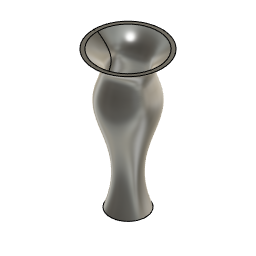
Vase v2 (Autodesk Fusion 360 design; units mm, degrees)
Autodesk Fusion 360 part; units mm, degrees
sketch "S-Vase-1" plane through (0, 0, 0) normal (0, 1, 0) x (1, 0, 0)
  line L0 (-88.461091, -147.362553) -> (-98.372625, -147.362553)
  spline S0 degree 5 poles (-98.372625, -147.362553) (-90.575572, -142.36067) (-76.825516, -132.431886) (-61.732191, -117.763849) (-51.958026, -98.828036) (-52.930643, -77.034995) (-62.024, -57.890704) (-74.243788, -41.693247) (-86.035966, -27.652867) (-95.531073, -13.982558) (-101.865459, 1.426054) (-104.795967, 20.4963) (-104.240926, 44.41601) (-100.243032, 73.849599) (-92.907373, 109.081445) (-82.364022, 150.155399) (-71.459298, 187.620816) (-61.929932, 218.259655) (-54.980996, 239.806153) (-51.35752, 250.859554) knots 0 0 0 0 0 0 0.06666667 0.13333333 0.2 0.26666667 0.33333333 0.4 0.46666667 0.53333333 0.6 0.66666667 0.73333333 0.8 0.86666667 0.93333333 1 1 1 1 1 1
  line L1 (-51.35752, 250.859554) -> (-0.678901, 250.859554)
  line L2 (-0.678901, 250.859554) -> (-0.453754, -147.362553)
  line L3 (-163.094718, -188.882386) -> (-33.650533, -105.84272)
  spline S1 degree 5 poles (-88.461091, -147.362553) (-80.720692, -142.397014) (-67.056368, -132.540065) (-52.008939, -117.977208) (-42.150348, -99.17113) (-42.881833, -77.499276) (-51.719986, -58.420857) (-63.770855, -42.243259) (-75.506283, -28.237163) (-85.061193, -14.682918) (-91.56478, 0.467783) (-94.773244, 19.11565) (-94.60872, 42.45327) (-91.110969, 71.147147) (-84.381692, 105.488788) (-74.546413, 145.528366) (-64.286411, 182.055738) (-55.283352, 211.930616) (-48.70416, 232.941151) (-45.270275, 243.719908) knots 0 0 0 0 0 0 0.06666667 0.13333333 0.2 0.26666667 0.33333333 0.4 0.46666667 0.53333333 0.6 0.66666667 0.73333333 0.8 0.86666667 0.93333333 1 1 1 1 1 1
  line L4 (-153.183183, -188.882386) -> (-23.738998, -105.84272)
  line L5 (-45.270275, 243.719908) -> (-0.674879, 243.745121)
  line L6 (-88.461091, -147.362553) -> (-98.372625, -147.362553)
  line L7 (-51.35752, 250.859554) -> (-0.678901, 250.859554)
  spline S2 degree 5 poles (-88.461091, -147.362553) (-80.720692, -142.397014) (-67.056368, -132.540065) (-52.008939, -117.977208) (-42.150348, -99.17113) (-42.881833, -77.499276) (-51.719986, -58.420857) (-63.770855, -42.243259) (-75.506283, -28.237163) (-85.061193, -14.682918) (-91.56478, 0.467783) (-94.773244, 19.11565) (-94.60872, 42.45327) (-91.110969, 71.147147) (-84.381692, 105.488788) (-74.546413, 145.528366) (-64.286411, 182.055738) (-55.283352, 211.930616) (-48.70416, 232.941151) (-45.270275, 243.719908) knots 0 0 0 0 0 0 0.06666667 0.13333333 0.2 0.26666667 0.33333333 0.4 0.46666667 0.53333333 0.6 0.66666667 0.73333333 0.8 0.86666667 0.93333333 1 1 1 1 1 1
  line L8 (-153.183183, -188.882386) -> (-23.738998, -105.84272)
  line L9 (-88.461091, -147.362553) -> (-98.372625, -147.362553)
  line L10 (-88.461091, -147.362553) -> (-98.372625, -147.362553)
  spline S3 degree 5 poles (-98.372625, -147.362553) (-90.575572, -142.36067) (-76.825516, -132.431886) (-61.732191, -117.763849) (-51.958026, -98.828036) (-52.930643, -77.034995) (-62.024, -57.890704) (-74.243788, -41.693247) (-86.035966, -27.652867) (-95.531073, -13.982558) (-101.865459, 1.426054) (-104.795967, 20.4963) (-104.240926, 44.41601) (-100.243032, 73.849599) (-92.907373, 109.081445) (-82.364022, 150.155399) (-71.459298, 187.620816) (-61.929932, 218.259655) (-54.980996, 239.806153) (-51.35752, 250.859554) knots 0 0 0 0 0 0 0.06666667 0.13333333 0.2 0.26666667 0.33333333 0.4 0.46666667 0.53333333 0.6 0.66666667 0.73333333 0.8 0.86666667 0.93333333 1 1 1 1 1 1
  line L11 (-163.094718, -188.882386) -> (-33.650533, -105.84272)
  line L12 (-0.678901, 250.859554) -> (-0.453754, -147.362553)
  line L13 (-45.270275, 243.719908) -> (-0.674879, 243.745121)
  spline S4 degree 5 poles (-88.461091, -147.362553) (-80.720692, -142.397014) (-67.056368, -132.540065) (-52.008939, -117.977208) (-42.150348, -99.17113) (-42.881833, -77.499276) (-51.719986, -58.420857) (-63.770855, -42.243259) (-75.506283, -28.237163) (-85.061193, -14.682918) (-91.56478, 0.467783) (-94.773244, 19.11565) (-94.60872, 42.45327) (-91.110969, 71.147147) (-84.381692, 105.488788) (-74.546413, 145.528366) (-64.286411, 182.055738) (-55.283352, 211.930616) (-48.70416, 232.941151) (-45.270275, 243.719908) knots 0 0 0 0 0 0 0.06666667 0.13333333 0.2 0.26666667 0.33333333 0.4 0.46666667 0.53333333 0.6 0.66666667 0.73333333 0.8 0.86666667 0.93333333 1 1 1 1 1 1
  line L14 (-153.183183, -188.882386) -> (-23.738998, -105.84272)
  line L15 (-0.678901, 250.859554) -> (-0.453754, -147.362553)
  line L16 (-51.35752, 250.859554) -> (-0.678901, 250.859554)
  line L17 (-45.270275, 243.719908) -> (-0.674879, 243.745121)
  line L18 (-51.35752, 250.859554) -> (-0.678901, 250.859554)
  line L19 (-45.270275, 243.719908) -> (-0.674879, 243.745121)
  line L20 (-0.678901, 250.859554) -> (-0.453754, -147.362553)
  spline S5 degree 5 poles (-98.372625, -147.362553) (-90.575572, -142.36067) (-76.825516, -132.431886) (-61.732191, -117.763849) (-51.958026, -98.828036) (-52.930643, -77.034995) (-62.024, -57.890704) (-74.243788, -41.693247) (-86.035966, -27.652867) (-95.531073, -13.982558) (-101.865459, 1.426054) (-104.795967, 20.4963) (-104.240926, 44.41601) (-100.243032, 73.849599) (-92.907373, 109.081445) (-82.364022, 150.155399) (-71.459298, 187.620816) (-61.929932, 218.259655) (-54.980996, 239.806153) (-51.35752, 250.859554) knots 0 0 0 0 0 0 0.06666667 0.13333333 0.2 0.26666667 0.33333333 0.4 0.46666667 0.53333333 0.6 0.66666667 0.73333333 0.8 0.86666667 0.93333333 1 1 1 1 1 1
  line L21 (-163.094718, -188.882386) -> (-33.650533, -105.84272)
  line L22 (-88.461091, -147.362553) -> (-98.372625, -147.362553)
  line L23 (-88.461091, -147.362553) -> (-98.372625, -147.362553)
  spline S6 degree 5 poles (-88.461091, -147.362553) (-80.720692, -142.397014) (-67.056368, -132.540065) (-52.008939, -117.977208) (-42.150348, -99.17113) (-42.881833, -77.499276) (-51.719986, -58.420857) (-63.770855, -42.243259) (-75.506283, -28.237163) (-85.061193, -14.682918) (-91.56478, 0.467783) (-94.773244, 19.11565) (-94.60872, 42.45327) (-91.110969, 71.147147) (-84.381692, 105.488788) (-74.546413, 145.528366) (-64.286411, 182.055738) (-55.283352, 211.930616) (-48.70416, 232.941151) (-45.270275, 243.719908) knots 0 0 0 0 0 0 0.06666667 0.13333333 0.2 0.26666667 0.33333333 0.4 0.46666667 0.53333333 0.6 0.66666667 0.73333333 0.8 0.86666667 0.93333333 1 1 1 1 1 1
  line L24 (-153.183183, -188.882386) -> (-23.738998, -105.84272)
  spline S7 degree 5 poles (-98.372625, -147.362553) (-90.575572, -142.36067) (-76.825516, -132.431886) (-61.732191, -117.763849) (-51.958026, -98.828036) (-52.930643, -77.034995) (-62.024, -57.890704) (-74.243788, -41.693247) (-86.035966, -27.652867) (-95.531073, -13.982558) (-101.865459, 1.426054) (-104.795967, 20.4963) (-104.240926, 44.41601) (-100.243032, 73.849599) (-92.907373, 109.081445) (-82.364022, 150.155399) (-71.459298, 187.620816) (-61.929932, 218.259655) (-54.980996, 239.806153) (-51.35752, 250.859554) knots 0 0 0 0 0 0 0.06666667 0.13333333 0.2 0.26666667 0.33333333 0.4 0.46666667 0.53333333 0.6 0.66666667 0.73333333 0.8 0.86666667 0.93333333 1 1 1 1 1 1
  line L25 (-163.094718, -188.882386) -> (-33.650533, -105.84272)
  line L26 (-88.461091, -147.362553) -> (-98.372625, -147.362553)
  line L27 (-88.461091, -147.362553) -> (-98.372625, -147.362553)
  line L28 (-51.35752, 250.859554) -> (-0.678901, 250.859554)
  spline S8 degree 5 poles (-88.461091, -147.362553) (-80.720692, -142.397014) (-67.056368, -132.540065) (-52.008939, -117.977208) (-42.150348, -99.17113) (-42.881833, -77.499276) (-51.719986, -58.420857) (-63.770855, -42.243259) (-75.506283, -28.237163) (-85.061193, -14.682918) (-91.56478, 0.467783) (-94.773244, 19.11565) (-94.60872, 42.45327) (-91.110969, 71.147147) (-84.381692, 105.488788) (-74.546413, 145.528366) (-64.286411, 182.055738) (-55.283352, 211.930616) (-48.70416, 232.941151) (-45.270275, 243.719908) knots 0 0 0 0 0 0 0.06666667 0.13333333 0.2 0.26666667 0.33333333 0.4 0.46666667 0.53333333 0.6 0.66666667 0.73333333 0.8 0.86666667 0.93333333 1 1 1 1 1 1
  line L29 (-153.183183, -188.882386) -> (-23.738998, -105.84272)
  line L30 (-51.35752, 250.859554) -> (-0.678901, 250.859554)
  line L31 (-88.461091, -147.362553) -> (-98.372625, -147.362553)
  line L32 (-0.678901, 250.859554) -> (-0.453754, -147.362553)
  spline S9 degree 5 poles (-98.372625, -147.362553) (-90.575572, -142.36067) (-76.825516, -132.431886) (-61.732191, -117.763849) (-51.958026, -98.828036) (-52.930643, -77.034995) (-62.024, -57.890704) (-74.243788, -41.693247) (-86.035966, -27.652867) (-95.531073, -13.982558) (-101.865459, 1.426054) (-104.795967, 20.4963) (-104.240926, 44.41601) (-100.243032, 73.849599) (-92.907373, 109.081445) (-82.364022, 150.155399) (-71.459298, 187.620816) (-61.929932, 218.259655) (-54.980996, 239.806153) (-51.35752, 250.859554) knots 0 0 0 0 0 0 0.06666667 0.13333333 0.2 0.26666667 0.33333333 0.4 0.46666667 0.53333333 0.6 0.66666667 0.73333333 0.8 0.86666667 0.93333333 1 1 1 1 1 1
  line L33 (-163.094718, -188.882386) -> (-33.650533, -105.84272)
  line L34 (-0.678901, 250.859554) -> (-0.453754, -147.362553)
  spline S10 degree 5 poles (-98.372625, -147.362553) (-90.575572, -142.36067) (-76.825516, -132.431886) (-61.732191, -117.763849) (-51.958026, -98.828036) (-52.930643, -77.034995) (-62.024, -57.890704) (-74.243788, -41.693247) (-86.035966, -27.652867) (-95.531073, -13.982558) (-101.865459, 1.426054) (-104.795967, 20.4963) (-104.240926, 44.41601) (-100.243032, 73.849599) (-92.907373, 109.081445) (-82.364022, 150.155399) (-71.459298, 187.620816) (-61.929932, 218.259655) (-54.980996, 239.806153) (-51.35752, 250.859554) knots 0 0 0 0 0 0 0.06666667 0.13333333 0.2 0.26666667 0.33333333 0.4 0.46666667 0.53333333 0.6 0.66666667 0.73333333 0.8 0.86666667 0.93333333 1 1 1 1 1 1
  line L35 (-163.094718, -188.882386) -> (-33.650533, -105.84272)
  line L36 (-45.270275, 243.719908) -> (-0.674879, 243.745121)
  spline S11 degree 5 poles (-88.461091, -147.362553) (-80.720692, -142.397014) (-67.056368, -132.540065) (-52.008939, -117.977208) (-42.150348, -99.17113) (-42.881833, -77.499276) (-51.719986, -58.420857) (-63.770855, -42.243259) (-75.506283, -28.237163) (-85.061193, -14.682918) (-91.56478, 0.467783) (-94.773244, 19.11565) (-94.60872, 42.45327) (-91.110969, 71.147147) (-84.381692, 105.488788) (-74.546413, 145.528366) (-64.286411, 182.055738) (-55.283352, 211.930616) (-48.70416, 232.941151) (-45.270275, 243.719908) knots 0 0 0 0 0 0 0.06666667 0.13333333 0.2 0.26666667 0.33333333 0.4 0.46666667 0.53333333 0.6 0.66666667 0.73333333 0.8 0.86666667 0.93333333 1 1 1 1 1 1
  line L37 (-153.183183, -188.882386) -> (-23.738998, -105.84272)
  line L38 (-88.461091, -147.362553) -> (-98.372625, -147.362553)
  line L39 (-88.461091, -147.362553) -> (-98.372625, -147.362553)
  line L40 (-51.35752, 250.859554) -> (-0.678901, 250.859554)
  line L41 (-88.461091, -147.362553) -> (-98.372625, -147.362553)
  spline S12 degree 5 poles (-98.372625, -147.362553) (-90.575572, -142.36067) (-76.825516, -132.431886) (-61.732191, -117.763849) (-51.958026, -98.828036) (-52.930643, -77.034995) (-62.024, -57.890704) (-74.243788, -41.693247) (-86.035966, -27.652867) (-95.531073, -13.982558) (-101.865459, 1.426054) (-104.795967, 20.4963) (-104.240926, 44.41601) (-100.243032, 73.849599) (-92.907373, 109.081445) (-82.364022, 150.155399) (-71.459298, 187.620816) (-61.929932, 218.259655) (-54.980996, 239.806153) (-51.35752, 250.859554) knots 0 0 0 0 0 0 0.06666667 0.13333333 0.2 0.26666667 0.33333333 0.4 0.46666667 0.53333333 0.6 0.66666667 0.73333333 0.8 0.86666667 0.93333333 1 1 1 1 1 1
  line L42 (-163.094718, -188.882386) -> (-33.650533, -105.84272)
  line L43 (-45.270275, 243.719908) -> (-0.674879, 243.745121)
  spline S13 degree 5 poles (-88.461091, -147.362553) (-80.720692, -142.397014) (-67.056368, -132.540065) (-52.008939, -117.977208) (-42.150348, -99.17113) (-42.881833, -77.499276) (-51.719986, -58.420857) (-63.770855, -42.243259) (-75.506283, -28.237163) (-85.061193, -14.682918) (-91.56478, 0.467783) (-94.773244, 19.11565) (-94.60872, 42.45327) (-91.110969, 71.147147) (-84.381692, 105.488788) (-74.546413, 145.528366) (-64.286411, 182.055738) (-55.283352, 211.930616) (-48.70416, 232.941151) (-45.270275, 243.719908) knots 0 0 0 0 0 0 0.06666667 0.13333333 0.2 0.26666667 0.33333333 0.4 0.46666667 0.53333333 0.6 0.66666667 0.73333333 0.8 0.86666667 0.93333333 1 1 1 1 1 1
  line L44 (-153.183183, -188.882386) -> (-23.738998, -105.84272)
  line L45 (-45.270275, 243.719908) -> (-0.674879, 243.745121)
  spline S14 degree 5 poles (-88.461091, -147.362553) (-80.720692, -142.397014) (-67.056368, -132.540065) (-52.008939, -117.977208) (-42.150348, -99.17113) (-42.881833, -77.499276) (-51.719986, -58.420857) (-63.770855, -42.243259) (-75.506283, -28.237163) (-85.061193, -14.682918) (-91.56478, 0.467783) (-94.773244, 19.11565) (-94.60872, 42.45327) (-91.110969, 71.147147) (-84.381692, 105.488788) (-74.546413, 145.528366) (-64.286411, 182.055738) (-55.283352, 211.930616) (-48.70416, 232.941151) (-45.270275, 243.719908) knots 0 0 0 0 0 0 0.06666667 0.13333333 0.2 0.26666667 0.33333333 0.4 0.46666667 0.53333333 0.6 0.66666667 0.73333333 0.8 0.86666667 0.93333333 1 1 1 1 1 1
  line L46 (-153.183183, -188.882386) -> (-23.738998, -105.84272)
  spline S15 degree 5 poles (-98.372625, -147.362553) (-90.575572, -142.36067) (-76.825516, -132.431886) (-61.732191, -117.763849) (-51.958026, -98.828036) (-52.930643, -77.034995) (-62.024, -57.890704) (-74.243788, -41.693247) (-86.035966, -27.652867) (-95.531073, -13.982558) (-101.865459, 1.426054) (-104.795967, 20.4963) (-104.240926, 44.41601) (-100.243032, 73.849599) (-92.907373, 109.081445) (-82.364022, 150.155399) (-71.459298, 187.620816) (-61.929932, 218.259655) (-54.980996, 239.806153) (-51.35752, 250.859554) knots 0 0 0 0 0 0 0.06666667 0.13333333 0.2 0.26666667 0.33333333 0.4 0.46666667 0.53333333 0.6 0.66666667 0.73333333 0.8 0.86666667 0.93333333 1 1 1 1 1 1
  line L47 (-163.094718, -188.882386) -> (-33.650533, -105.84272)
  line L48 (-45.270275, 243.719908) -> (-0.674879, 243.745121)
  line L49 (-88.461091, -147.362553) -> (-98.372625, -147.362553)
  line L50 (-51.35752, 250.859554) -> (-0.678901, 250.859554)
  line L51 (-88.461091, -147.362553) -> (-98.372625, -147.362553)
  line L52 (-88.461091, -147.362553) -> (-98.372625, -147.362553)
  line L53 (-88.461091, -147.362553) -> (-98.372625, -147.362553)
  line L54 (-0.678901, 250.859554) -> (-0.453754, -147.362553)
  line L55 (-0.678901, 250.859554) -> (-0.453754, -147.362553)
  point P0 (-67.843336, -50.76982)
  point P1 (-100.780848, 1.471904)
  point P2 (-57.843336, -50.76982)
  point P3 (-90.780848, 1.471904)
  point P4 (-0.674879, 243.745121)
  point P5 (-88.461091, -147.362553)
  point P6 (-57.843336, -50.76982)
  point P7 (-0.674879, 243.745121)
  point P8 (-90.780848, 1.471904)
  point P9 (-88.461091, -147.362553)
  point P10 (-67.843336, -50.76982)
  point P11 (-100.780848, 1.471904)
  point P12 (-90.780848, 1.471904)
  point P13 (-57.843336, -50.76982)
  point P14 (-0.674879, 243.745121)
  point P15 (-88.461091, -147.362553)
  point P16 (-67.843336, -50.76982)
  point P17 (-0.674879, 243.745121)
  point P18 (-90.780848, 1.471904)
  point P19 (-88.461091, -147.362553)
  point P20 (-57.843336, -50.76982)
  point P21 (-67.843336, -50.76982)
  point P22 (-100.780848, 1.471904)
  point P23 (-100.780848, 1.471904)
  point P24 (-88.461091, -147.362553)
  point P25 (-88.461091, -147.362553)
  point P26 (-90.780848, 1.471904)
  point P27 (-88.461091, -147.362553)
  point P28 (-67.843336, -50.76982)
  point P29 (-100.780848, 1.471904)
  point P30 (-0.674879, 243.745121)
  point P31 (-0.674879, 243.745121)
  point P32 (-57.843336, -50.76982)
  point P33 (-57.843336, -50.76982)
  point P34 (-67.843336, -50.76982)
  point P35 (-57.843336, -50.76982)
  point P36 (-67.843336, -50.76982)
  point P37 (-90.780848, 1.471904)
  point P38 (-0.674879, 243.745121)
  point P39 (-90.780848, 1.471904)
  point P40 (-57.843336, -50.76982)
  point P41 (-100.780848, 1.471904)
  point P42 (-100.780848, 1.471904)
  point P43 (-0.674879, 243.745121)
  point P44 (-90.780848, 1.471904)
  point P45 (-88.461091, -147.362553)
  point P46 (-67.843336, -50.76982)
  point P47 (-100.780848, 1.471904)
  constraint horizontal L0
  constraint horizontal L1
  constraint perpendicular L2 L5
  constraint parallel L0 L6
  constraint horizontal L10
  constraint horizontal L7
  constraint perpendicular L12 L13
  constraint parallel L9 L10
  constraint horizontal L27
  constraint horizontal L16
  constraint perpendicular L17 L20
  constraint parallel L26 L27
  constraint horizontal L23
  constraint horizontal L18
  constraint perpendicular L15 L19
  constraint parallel L22 L23
  constraint horizontal L52
  constraint horizontal L28
  constraint perpendicular L45 L54
  constraint parallel L51 L52
  constraint horizontal L53
  constraint horizontal L30
  constraint perpendicular L43 L55
  constraint parallel L49 L53
  constraint horizontal L39
  constraint horizontal L50
  constraint perpendicular L34 L36
  constraint parallel L31 L39
  constraint horizontal L38
  constraint horizontal L40
  constraint perpendicular L32 L48
  constraint parallel L38 L41
revolve "Revolve1" add sketch "S-Vase-1" angle 360 about axis through (-0.678901, 0, -250.859554) along (0.00056538, 0, 0.99999984) contours L0 L3 S1 L6 S2 L9 L10 L11 S4 L21 L22 L23 S6 L25 L26 L27 S8 L31 L33 L35 S11 L38 L39 L41 L42 S13 S14 L47 L49 L51 L52 L53 | S0 L1 L2 L3 S1 L5 L7 S2 S3 L11 L12 L13 S4 L15 L16 L17 L18 L19 L20 S5 L21 S6 S7 L25 L28 S8 L30 L32 S9 L33 L34 S10 L35 L36 S11 L40 S12 L42 L43 S13 L45 S14 S15 L47 L48 L50 L54 L55 picked at (-86.207246, -143.369918) picked at (-89.750825, 88.062526) makes body 1
sketch "S-Vase-2" plane through (0, 0, 0) normal (0, 1, 0) x (1, 0, 0)
  line L0 (-51.69142, 250.516486) -> (-0.097963, 250.858791)
  spline S0 degree 5 poles (-88.861253, -147.663022) (-81.087174, -142.468117) (-67.6242, -132.328566) (-53.684568, -117.869953) (-46.444116, -99.970291) (-49.850564, -79.185234) (-58.014232, -59.091896) (-63.963404, -38.785179) (-64.048284, -17.580634) (-58.118349, 4.943825) (-48.016612, 29.034221) (-36.658752, 54.799773) (-26.914793, 82.261958) (-20.628361, 111.390198) (-18.876176, 142.126502) (-22.179255, 174.404369) (-28.994921, 201.412062) (-36.442386, 222.315816) (-42.437945, 236.537559) (-45.693372, 243.719908) knots 0 0 0 0 0 0 0.06666667 0.13333333 0.2 0.26666667 0.33333333 0.4 0.46666667 0.53333333 0.6 0.66666667 0.73333333 0.8 0.86666667 0.93333333 1 1 1 1 1 1
  line L1 (-152.806961, -190.393727) -> (-24.915544, -104.932318)
  line L2 (-0.097963, 250.859621) -> (-0.097963, -147.362542)
  spline S1 degree 5 poles (-99.065951, -147.663022) (-91.10644, -142.567056) (-77.279413, -132.617683) (-62.814185, -118.421207) (-54.954296, -100.784053) (-57.935381, -79.971468) (-66.249603, -59.275673) (-73.087588, -37.651102) (-74.770419, -14.474195) (-70.797782, 10.441894) (-62.55988, 37.017474) (-52.51751, 65.007848) (-43.289639, 94.116966) (-36.684247, 124.10986) (-33.742393, 154.821752) (-34.995663, 186.142291) (-39.495721, 211.634626) (-44.835229, 230.985951) (-49.261573, 243.98924) (-51.69142, 250.516486) knots 0 0 0 0 0 0 0.06666667 0.13333333 0.2 0.26666667 0.33333333 0.4 0.46666667 0.53333333 0.6 0.66666667 0.73333333 0.8 0.86666667 0.93333333 1 1 1 1 1 1
  line L3 (-163.825522, -189.124437) -> (-34.30638, -106.201608)
  line L4 (-45.693372, 243.719908) -> (-0.097963, 243.719908)
  line L5 (-99.065951, -147.663022) -> (-88.861253, -147.663022)
  spline S2 degree 5 poles (-98.579966, -147.351055) (-98.579966, -147.351054) (-98.579966, -147.351054) (-98.579965, -147.351054) (-98.579965, -147.351053) (-98.579965, -147.351053) knots 0.99998931 0.99998931 0.99998931 0.99998931 0.99998931 0.99998931 1 1 1 1 1 1
  point P0 (-68.449487, -51.097884)
  point P1 (-37.422993, 54.277633)
  point P2 (-51.009044, 70.494636)
  point P3 (-0.423097, 0)
  point P4 (-60.05539, -50.514552)
  point P5 (-0.423097, 0)
  constraint horizontal L5
  constraint perpendicular L2 L4
  constraint horizontal L4
revolve "Revolve2" add sketch "S-Vase-2" angle 360 about axis through (-0.097963, 0, -250.859621) along (0, 0, 1) separate body contours L0 S0 L2 S1 L3 L4 | S0 S1 L3 L5 picked at (-44.994356, 71.168327) picked at (-86.971819, -143.748141) makes body 2
hidden bodies 1
named bodies: "Vase-1", "Vase-2"
